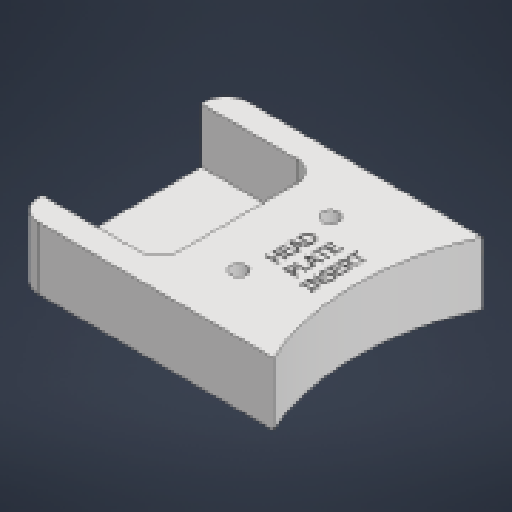
# Autodesk Inventor part: Head Plate Inserts
Saved by Autodesk Inventor 2026.1 (Build 301233000, 233)
## iProperties
Created: 2025-06-24
Part Number: Head Plate Inserts
Material: Generic
Document SubType Name: Modeling
Designer: mumin
Density: 1 g/cm^3
Appearance: Default
Author: mumin
Autodesk Inventor part; units mm, degrees
note: some values were not read from the file. Chosen so that the rebuilt part matches the saved one: direction of "Hole1".
ref_plane "YZ Plane" through (0, 0, 0) normal (1, 0, 0) x (0, 1, 0)
ref_plane "XZ Plane" through (0, 0, 0) normal (0, 1, 0) x (-1, 0, 0)
sketch "Sketch1" plane through (0, 0, 0) normal (0, 1, 0) x (-1, 0, 0)
  circle A0 centre (0, 0) radius 42.5
  arc A1 (55.6417, 25) -> (-59.6645, -12.6946) centre (0, 0) ccw
  line L0 (0, 0) -> (0, -61)
  line L1 (0, 0) -> (0, 0)
  line L2 (117.5, -25) -> (117.5, 25)
  line L3 (117.5, 25) -> (-117.5, -25) construction
  line L4 (-117.5, 25) -> (117.5, -25) construction
  line L5 (117.5, 25) -> (55.6417, 25)
  line L6 (55.6417, -25) -> (117.5, -25)
  arc A2 (-59.6645, -12.6946) -> (55.6417, -25) centre (0, 0) ccw
  point P0 (0, -61)
  point P1 (-59.6645, 12.6946)
  dimension "d0" = 85
  dimension "d1" = 61
  dimension "d2" = 235
  constraints: 14 end point, 5 coincident, 5 point on circle, 3 centre point, 2 horizontal, 2 midpoint, 2 point on line, 1 parallel, 1 vertical, 1 vertical alignment
  measures "d0" diameter of A0
  measures "d1" radius of A1
  measures "d2" distance of L4.end L3.end
extrude "Head Plate Geometry" add sketch "Sketch1" along normal blind 15
sketch "Sketch2" plane through (0, 15, 0) normal (0, 1, 0) x (1, 0, 0)
  line L0 (-117.5, 25) -> (-117.5, -25) projected
  line L1 (-117.5, 19) -> (-94.5, 19)
  line L2 (-89.5, 14) -> (-89.5, -14)
  line L3 (-94.5, -19) -> (-117.5, -19)
  arc A0 (-89.5, 14) -> (-94.5, 19) centre (-94.5, 14) ccw
  arc A1 (-94.5, -19) -> (-89.5, -14) centre (-94.5, -14) ccw
  line L4 (-117.5, 25) -> (-117.5, -25) projected
  line L5 (-153.2, 0) -> (96.7, 0) projected
  point P0 (0, 0)
  dimension "d6" = 5
  dimension "d7" = 38
  dimension "d8" = 28
  constraints: 6 end point, 4 point on circle, 4 tangent, 2 centre point, 2 perpendicular, 2 point on line, 1 equal radius, 1 horizontal, 1 other
  measures "d6" radius of A0
  measures "d7" distance between parallel lines of L3 L1
  measures "d8" distance between parallel lines of L2 L0
extrude "Magnet Seat" cut sketch "Sketch2" against normal blind 13.1
sketch "Sketch3" plane through (0, 0, 0) normal (0, -1, 0) x (1, 0, 0)
  line L0 (-117.5, -25) -> (-117.5, 25) projected
  line L1 (-153.2, 0) -> (96.7, 0) projected
  point P0 (0, 0)
  point P1 (-78.5, -11)
  point P2 (-78.5, 11)
  dimension "d19" = 39
  dimension "d22" = 11
  constraints: 1 symmetric about line
  measures "d19" distance from line of L0 point (-78.5, -11)
  measures "d22" distance from line of L1 point (-78.5, -11)
hole "Hole1" at (-78.5, 0, -11) at (-78.5, 0, 11) direction (0, 1, 0) diameter 4 depth 15 counterbore diameter 8 counterbore depth 6
fillet "Fillet1" radius 5 2 edges at (-117.5, 7.5, -25) (-117.5, 7.5, 25)
sketch "Sketch4" plane through (0, 0, 0) normal (0, -1, 0) x (1, 0, 0)
  circle A0 centre (0, 0) radius 61.5
  dimension "d24" = 123
  constraints: 1 centre point, 1 coincident
  measures "d24" diameter of A0
extrude "Remove Material" cut sketch "Sketch4" against normal through all
sketch "Sketch5" plane through (0, 15, 0) normal (0, 1, 0) x (1, 0, 0)
  line L0 (-78.3069, -19.4191) -> (-78.3069, 19.5479) construction
  line L1 (-78.3069, 19.5479) -> (-42.2723, 19.5479) construction
  line L2 (-42.2723, 19.5479) -> (-42.2723, -19.4191) construction
  line L3 (-42.2723, -19.4191) -> (-78.3069, -19.4191) construction
  line L4 (-75.2589, -2.6835) -> (-75.2589, -3.0886)
  line L5 (-75.2589, -3.0886) -> (-76.7507, -3.0886)
  line L6 (-76.7507, -3.0886) -> (-76.7507, -4.4916)
  line L7 (-76.7507, -4.4916) -> (-75.2589, -4.4916)
  line L8 (-75.2589, -4.4916) -> (-75.2589, -4.8967)
  line L9 (-75.2589, -4.8967) -> (-78.3069, -4.8967)
  line L10 (-78.3069, -4.8967) -> (-78.3069, -4.4916)
  line L11 (-78.3069, -4.4916) -> (-77.1114, -4.4916)
  line L12 (-77.1114, -4.4916) -> (-77.1114, -3.0886)
  line L13 (-77.1114, -3.0886) -> (-78.3069, -3.0886)
  line L14 (-78.3069, -3.0886) -> (-78.3069, -2.6835)
  line L15 (-78.3069, -2.6835) -> (-75.2589, -2.6835)
  line L16 (-75.2589, -2.066) -> (-78.3069, -2.066)
  line L17 (-78.3069, -2.066) -> (-78.3069, -0.1592)
  line L18 (-78.3069, -0.1592) -> (-77.9462, -0.1592)
  line L19 (-77.9462, -0.1592) -> (-77.9462, -1.6609)
  line L20 (-77.9462, -1.6609) -> (-77.1114, -1.6609)
  line L21 (-77.1114, -1.6609) -> (-77.1114, -0.2604)
  line L22 (-77.1114, -0.2604) -> (-76.7507, -0.2604)
  line L23 (-76.7507, -0.2604) -> (-76.7507, -1.6609)
  line L24 (-76.7507, -1.6609) -> (-75.6195, -1.6609)
  line L25 (-75.6195, -1.6609) -> (-75.6195, -0.1592)
  line L26 (-75.6195, -0.1592) -> (-75.2589, -0.1592)
  line L27 (-75.2589, -0.1592) -> (-75.2589, -2.066)
  line L28 (-75.2589, -0.0431) -> (-78.3069, 0.9844)
  line L29 (-78.3069, 0.9844) -> (-78.3069, 1.4834)
  line L30 (-78.3069, 1.4834) -> (-75.2589, 2.5109)
  line L31 (-75.2589, 2.5109) -> (-75.2589, 2.0836)
  line L32 (-75.2589, 2.0836) -> (-76.111, 1.807)
  line L33 (-76.111, 1.807) -> (-76.111, 0.6436)
  line L34 (-76.111, 0.6436) -> (-75.2589, 0.3669)
  line L35 (-75.2589, 0.3669) -> (-75.2589, -0.0431)
  line L36 (-76.4568, 1.6958) -> (-77.8919, 1.224)
  line L37 (-77.8919, 1.224) -> (-76.4568, 0.7547)
  line L38 (-76.4568, 0.7547) -> (-76.4568, 1.6958)
  spline S0 degree 2 poles (-76.7804, 5.2032) (-76.363, 5.2032) (-75.6911, 4.8648) (-75.5034, 4.5808) knots 0 0 0 1 2 2 2
  spline S1 degree 2 poles (-75.5034, 4.5808) (-75.3577, 4.3486) (-75.2589, 3.8719) (-75.2589, 3.5014) knots 0 0 0 1 2 2 2
  line L39 (-75.2589, 3.5014) -> (-75.2589, 2.7999)
  line L40 (-75.2589, 2.7999) -> (-78.3069, 2.7999)
  line L41 (-78.3069, 2.7999) -> (-78.3069, 3.494)
  spline S2 degree 2 poles (-78.3069, 3.494) (-78.3069, 3.9238) (-78.1784, 4.4128) (-78.0648, 4.5857) knots 0 0 0 1 2 2 2
  spline S3 degree 2 poles (-78.0648, 4.5857) (-77.8697, 4.8797) (-77.225, 5.2032) (-76.7804, 5.2032) knots 0 0 0 1 2 2 2
  spline S4 degree 2 poles (-76.7853, 4.7809) (-77.1361, 4.7809) (-77.6325, 4.5487) (-77.7733, 4.319) knots 0 0 0 1 2 2 2
  spline S5 degree 2 poles (-77.7733, 4.319) (-77.8697, 4.1559) (-77.9561, 3.7879) (-77.9561, 3.5137) knots 0 0 0 1 2 2 2
  line L42 (-77.9561, 3.5137) -> (-77.9561, 3.205)
  line L43 (-77.9561, 3.205) -> (-75.6096, 3.205)
  line L44 (-75.6096, 3.205) -> (-75.6096, 3.5137)
  spline S6 degree 2 poles (-75.6096, 3.5137) (-75.6096, 3.783) (-75.6961, 4.1905) (-75.8121, 4.356) knots 0 0 0 1 2 2 2
  spline S7 degree 2 poles (-75.8121, 4.356) (-75.9554, 4.5684) (-76.4296, 4.7809) (-76.7853, 4.7809) knots 0 0 0 1 2 2 2
  spline S8 degree 2 poles (-72.3696, -3.5554) (-72.172, -3.5554) (-71.8163, -3.6962) (-71.6928, -3.8222) knots 0 0 0 1 2 2 2
  spline S9 degree 2 poles (-71.6928, -3.8222) (-71.5372, -3.9803) (-71.3766, -4.4076) (-71.3766, -4.7336) knots 0 0 0 1 2 2 2
  line L45 (-71.3766, -4.7336) -> (-71.3766, -5.077)
  line L46 (-71.3766, -5.077) -> (-70.2404, -5.077)
  line L47 (-70.2404, -5.077) -> (-70.2404, -5.4821)
  line L48 (-70.2404, -5.4821) -> (-73.2884, -5.4821)
  line L49 (-73.2884, -5.4821) -> (-73.2884, -4.7163)
  spline S10 degree 2 poles (-73.2884, -4.7163) (-73.2884, -4.4446) (-73.1995, -4.0643) (-73.0982, -3.9185) knots 0 0 0 1 2 2 2
  spline S11 degree 2 poles (-73.0982, -3.9185) (-72.9821, -3.7481) (-72.624, -3.5554) (-72.3696, -3.5554) knots 0 0 0 1 2 2 2
  spline S12 degree 2 poles (-72.3572, -3.9778) (-72.5153, -3.9778) (-72.7475, -4.0865) (-72.8216, -4.1976) knots 0 0 0 1 2 2 2
  spline S13 degree 2 poles (-72.8216, -4.1976) (-72.8858, -4.294) (-72.9377, -4.5509) (-72.9377, -4.741) knots 0 0 0 1 2 2 2
  line L50 (-72.9377, -4.741) -> (-72.9377, -5.077)
  line L51 (-72.9377, -5.077) -> (-71.7224, -5.077)
  line L52 (-71.7224, -5.077) -> (-71.7224, -4.8003)
  spline S14 degree 2 poles (-71.7224, -4.8003) (-71.7224, -4.5533) (-71.8015, -4.2495) (-71.9052, -4.1507) knots 0 0 0 1 2 2 2
  spline S15 degree 2 poles (-71.9052, -4.1507) (-71.9966, -4.0593) (-72.2115, -3.9778) (-72.3572, -3.9778) knots 0 0 0 1 2 2 2
  line L53 (-70.2404, -1.4041) -> (-70.2404, -3.1701)
  line L54 (-70.2404, -3.1701) -> (-73.2884, -3.1701)
  line L55 (-73.2884, -3.1701) -> (-73.2884, -2.765)
  line L56 (-73.2884, -2.765) -> (-70.601, -2.765)
  line L57 (-70.601, -2.765) -> (-70.601, -1.4041)
  line L58 (-70.601, -1.4041) -> (-70.2404, -1.4041)
  line L59 (-70.2404, -1.4139) -> (-73.2884, -0.3864)
  line L60 (-73.2884, -0.3864) -> (-73.2884, 0.1125)
  line L61 (-73.2884, 0.1125) -> (-70.2404, 1.1401)
  line L62 (-70.2404, 1.1401) -> (-70.2404, 0.7127)
  line L63 (-70.2404, 0.7127) -> (-71.0926, 0.4361)
  line L64 (-71.0926, 0.4361) -> (-71.0926, -0.7273)
  line L65 (-71.0926, -0.7273) -> (-70.2404, -1.0039)
  line L66 (-70.2404, -1.0039) -> (-70.2404, -1.4139)
  line L67 (-71.4384, 0.325) -> (-72.8734, -0.1468)
  line L68 (-72.8734, -0.1468) -> (-71.4384, -0.6161)
  line L69 (-71.4384, -0.6161) -> (-71.4384, 0.325)
  line L70 (-70.2404, 2.1404) -> (-72.9278, 2.1404)
  line L71 (-72.9278, 2.1404) -> (-72.9278, 1.1178)
  line L72 (-72.9278, 1.1178) -> (-73.2884, 1.1178)
  line L73 (-73.2884, 1.1178) -> (-73.2884, 3.5681)
  line L74 (-73.2884, 3.5681) -> (-72.9278, 3.5681)
  line L75 (-72.9278, 3.5681) -> (-72.9278, 2.5455)
  line L76 (-72.9278, 2.5455) -> (-70.2404, 2.5455)
  line L77 (-70.2404, 2.5455) -> (-70.2404, 2.1404)
  line L78 (-70.2404, 3.8768) -> (-73.2884, 3.8768)
  line L79 (-73.2884, 3.8768) -> (-73.2884, 5.7837)
  line L80 (-73.2884, 5.7837) -> (-72.9278, 5.7837)
  line L81 (-72.9278, 5.7837) -> (-72.9278, 4.2819)
  line L82 (-72.9278, 4.2819) -> (-72.0929, 4.2819)
  line L83 (-72.0929, 4.2819) -> (-72.0929, 5.6824)
  line L84 (-72.0929, 5.6824) -> (-71.7323, 5.6824)
  line L85 (-71.7323, 5.6824) -> (-71.7323, 4.2819)
  line L86 (-71.7323, 4.2819) -> (-70.601, 4.2819)
  line L87 (-70.601, 4.2819) -> (-70.601, 5.7837)
  line L88 (-70.601, 5.7837) -> (-70.2404, 5.7837)
  line L89 (-70.2404, 5.7837) -> (-70.2404, 3.8768)
  line L90 (-65.222, -5.6142) -> (-65.222, -6.7949)
  line L91 (-65.222, -6.7949) -> (-65.5332, -6.7949)
  line L92 (-65.5332, -6.7949) -> (-65.5332, -6.4071)
  line L93 (-65.5332, -6.4071) -> (-67.9587, -6.4071)
  line L94 (-67.9587, -6.4071) -> (-67.9587, -6.7949)
  line L95 (-67.9587, -6.7949) -> (-68.27, -6.7949)
  line L96 (-68.27, -6.7949) -> (-68.27, -5.6142)
  line L97 (-68.27, -5.6142) -> (-67.9587, -5.6142)
  line L98 (-67.9587, -5.6142) -> (-67.9587, -6.002)
  line L99 (-67.9587, -6.002) -> (-65.5332, -6.002)
  line L100 (-65.5332, -6.002) -> (-65.5332, -5.6142)
  line L101 (-65.5332, -5.6142) -> (-65.222, -5.6142)
  line L102 (-65.222, -2.9318) -> (-65.222, -3.3862)
  line L103 (-65.222, -3.3862) -> (-67.8501, -4.7349)
  line L104 (-67.8501, -4.7349) -> (-65.222, -4.7349)
  line L105 (-65.222, -4.7349) -> (-65.222, -5.1128)
  line L106 (-65.222, -5.1128) -> (-68.27, -5.1128)
  line L107 (-68.27, -5.1128) -> (-68.27, -4.5373)
  line L108 (-68.27, -4.5373) -> (-65.8567, -3.3097)
  line L109 (-65.8567, -3.3097) -> (-68.27, -3.3097)
  line L110 (-68.27, -3.3097) -> (-68.27, -2.9318)
  line L111 (-68.27, -2.9318) -> (-65.222, -2.9318)
  spline S16 degree 2 poles (-65.1676, -1.4646) (-65.1676, -1.7956) (-65.3059, -2.2599) (-65.4047, -2.4649) knots 0 0 0 1 2 2 2
  line L112 (-65.4047, -2.4649) -> (-65.9136, -2.4649)
  line L113 (-65.9136, -2.4649) -> (-65.9136, -2.4353)
  spline S17 degree 2 poles (-65.9136, -2.4353) (-65.7258, -2.2352) (-65.5184, -1.7289) (-65.5184, -1.4942) knots 0 0 0 1 2 2 2
  spline S18 degree 2 poles (-65.5184, -1.4942) (-65.5184, -1.1583) (-65.7975, -0.815) (-66.0272, -0.815) knots 0 0 0 1 2 2 2
  spline S19 degree 2 poles (-66.0272, -0.815) (-66.21, -0.815) (-66.4372, -0.9953) (-66.494, -1.1904) knots 0 0 0 1 2 2 2
  spline S20 degree 2 poles (-66.494, -1.1904) (-66.5335, -1.3312) (-66.5879, -1.5658) (-66.6323, -1.7412) knots 0 0 0 1 2 2 2
  spline S21 degree 2 poles (-66.6323, -1.7412) (-66.6743, -1.8993) (-66.8003, -2.1488) (-66.9016, -2.2451) knots 0 0 0 1 2 2 2
  spline S22 degree 2 poles (-66.9016, -2.2451) (-67.0028, -2.339) (-67.2745, -2.4427) (-67.4524, -2.4427) knots 0 0 0 1 2 2 2
  spline S23 degree 2 poles (-67.4524, -2.4427) (-67.8229, -2.4427) (-68.3243, -1.8647) (-68.3243, -1.4176) knots 0 0 0 1 2 2 2
  spline S24 degree 2 poles (-68.3243, -1.4176) (-68.3243, -1.1608) (-68.223, -0.7063) (-68.1267, -0.5111) knots 0 0 0 1 2 2 2
  line L114 (-68.1267, -0.5111) -> (-67.6426, -0.5111)
  line L115 (-67.6426, -0.5111) -> (-67.6426, -0.5408)
  spline S25 degree 2 poles (-67.6426, -0.5408) (-67.776, -0.6865) (-67.9736, -1.141) (-67.9736, -1.3905) knots 0 0 0 1 2 2 2
  spline S26 degree 2 poles (-67.9736, -1.3905) (-67.9736, -1.6721) (-67.7093, -2.0203) (-67.4944, -2.0203) knots 0 0 0 1 2 2 2
  spline S27 degree 2 poles (-67.4944, -2.0203) (-67.3017, -2.0203) (-67.072, -1.8153) (-67.0201, -1.6227) knots 0 0 0 1 2 2 2
  spline S28 degree 2 poles (-67.0201, -1.6227) (-66.9855, -1.4942) (-66.8966, -1.1212) (-66.8596, -0.9977) knots 0 0 0 1 2 2 2
  spline S29 degree 2 poles (-66.8596, -0.9977) (-66.7632, -0.684) (-66.3755, -0.3926) (-66.0914, -0.3926) knots 0 0 0 1 2 2 2
  spline S30 degree 2 poles (-66.0914, -0.3926) (-65.9111, -0.3926) (-65.5653, -0.5383) (-65.4443, -0.6692) knots 0 0 0 1 2 2 2
  spline S31 degree 2 poles (-65.4443, -0.6692) (-65.3109, -0.815) (-65.1676, -1.1855) (-65.1676, -1.4646) knots 0 0 0 1 2 2 2
  line L116 (-65.222, 0.0199) -> (-68.27, 0.0199)
  line L117 (-68.27, 0.0199) -> (-68.27, 1.9268)
  line L118 (-68.27, 1.9268) -> (-67.9093, 1.9268)
  line L119 (-67.9093, 1.9268) -> (-67.9093, 0.425)
  line L120 (-67.9093, 0.425) -> (-67.0745, 0.425)
  line L121 (-67.0745, 0.425) -> (-67.0745, 1.8255)
  line L122 (-67.0745, 1.8255) -> (-66.7138, 1.8255)
  line L123 (-66.7138, 1.8255) -> (-66.7138, 0.425)
  line L124 (-66.7138, 0.425) -> (-65.5826, 0.425)
  line L125 (-65.5826, 0.425) -> (-65.5826, 1.9268)
  line L126 (-65.5826, 1.9268) -> (-65.222, 1.9268)
  line L127 (-65.222, 1.9268) -> (-65.222, 0.0199)
  line L128 (-65.222, 4.7302) -> (-65.222, 4.2041)
  line L129 (-65.222, 4.2041) -> (-66.4347, 3.2408)
  line L130 (-66.4347, 3.2408) -> (-66.4347, 2.7764)
  line L131 (-66.4347, 2.7764) -> (-65.222, 2.7764)
  line L132 (-65.222, 2.7764) -> (-65.222, 2.3714)
  line L133 (-65.222, 2.3714) -> (-68.27, 2.3714)
  line L134 (-68.27, 2.3714) -> (-68.27, 3.1568)
  spline S32 degree 2 poles (-68.27, 3.1568) (-68.27, 3.4186) (-68.2131, 3.7719) (-68.1094, 3.9324) knots 0 0 0 1 2 2 2
  spline S33 degree 2 poles (-68.1094, 3.9324) (-68.0057, 4.093) (-67.6821, 4.2782) (-67.4425, 4.2782) knots 0 0 0 1 2 2 2
  spline S34 degree 2 poles (-67.4425, 4.2782) (-67.109, 4.2782) (-66.657, 3.9374) (-66.5484, 3.6459) knots 0 0 0 1 2 2 2
  line L135 (-66.5484, 3.6459) -> (-65.222, 4.7302)
  spline S35 degree 2 poles (-67.4104, 3.8558) (-67.5438, 3.8558) (-67.7488, 3.762) (-67.8155, 3.6632) knots 0 0 0 1 2 2 2
  spline S36 degree 2 poles (-67.8155, 3.6632) (-67.8723, 3.5767) (-67.9192, 3.347) (-67.9192, 3.1791) knots 0 0 0 1 2 2 2
  line L136 (-67.9192, 3.1791) -> (-67.9192, 2.7764)
  line L137 (-67.9192, 2.7764) -> (-66.7731, 2.7764)
  line L138 (-66.7731, 2.7764) -> (-66.7731, 3.1321)
  spline S37 degree 2 poles (-66.7731, 3.1321) (-66.7731, 3.3075) (-66.8349, 3.5866) (-66.9312, 3.6829) knots 0 0 0 1 2 2 2
  spline S38 degree 2 poles (-66.9312, 3.6829) (-67.0152, 3.7719) (-67.2523, 3.8558) (-67.4104, 3.8558) knots 0 0 0 1 2 2 2
  line L139 (-65.222, 5.6837) -> (-67.9093, 5.6837)
  line L140 (-67.9093, 5.6837) -> (-67.9093, 4.6611)
  line L141 (-67.9093, 4.6611) -> (-68.27, 4.6611)
  line L142 (-68.27, 4.6611) -> (-68.27, 7.1113)
  line L143 (-68.27, 7.1113) -> (-67.9093, 7.1113)
  line L144 (-67.9093, 7.1113) -> (-67.9093, 6.0887)
  line L145 (-67.9093, 6.0887) -> (-65.222, 6.0887)
  line L146 (-65.222, 6.0887) -> (-65.222, 5.6837)
  point P0 (0, 0)
  constraints: 2 other
emboss "Emboss1" sketch "Sketch5" operation cut depth 1 direction (0, -1, 0)
sketch "Sketch7" plane through (-112.5, 0, -25) normal (0, 0, -1) x (-1, 0, 0)
  line L0 (-47.4622, 6) -> (-53.4622, 6)
  line L1 (-53.4622, 12) -> (-53.4622, 6)
  line L2 (-47.4622, 12) -> (-53.4622, 12)
  line L3 (-47.4622, 6) -> (-47.4622, 12)
  line L4 (-53.4122, 6) -> (-53.4122, 12)
  line L5 (-47.5122, 6) -> (-47.5122, 12)
  line L6 (-53.4622, 11.95) -> (-47.4622, 11.95)
  line L7 (-53.4622, 6.05) -> (-47.4622, 6.05)
  point P0 (-112.5, 0)
  point P1 (-53.4122, 6.05)
  point P2 (-47.5122, 6.05)
  point P3 (-47.5122, 11.95)
  point P4 (-53.4122, 11.95)
  dimension "d57" = 0.05
  dimension "d58" = 0.05
  dimension "d59" = 0.05
  dimension "d60" = 0.05
  constraints: 16 end point, 8 point on line, 4 perpendicular, 2 horizontal, 2 vertical, 4 other
  measures "d57" distance between parallel lines of L3 L5
  measures "d58" distance between parallel lines of L1 L4
  measures "d59" distance between parallel lines of L2 L6
  measures "d60" distance between parallel lines of L0 L7
extrude "Catch" add sketch "Sketch7" along normal blind 3 contours L7 L4 L6 L5
chamfer "Chamfer7" distance 2.8 angle 45 2 edges at (-62.0378, 11.95, -28) (-62.0378, 6.05, -28) measured on face at (-63.0211, 8.0167, -28)
mirror "Mirror5" about plane through (0, 0, 0) normal (0, 0, 1) of "Catch", "Chamfer7"
body "Solid1"
